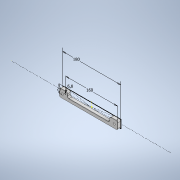
# Autodesk Inventor part: DisplayHolder
Saved by Autodesk Inventor 2022 (Build 260153000, 153)
## iProperties
Created: 2021-04-23
Part Number: DisplayHolder
Material: Generic
Document SubType Name: Modeling
Designer: Viktor
Density: 1 g/cm^3
Appearance: Default
Author: Viktor
## iProperties of the stored document DisplayHolder_3DPrint.ipt
Created: 2021-04-23
Part Number: DisplayHolder_3DPrint
Material: Generic
Document SubType Name: Modeling
Designer: Viktor
Density: 1 g/cm^3
Appearance: Default
Author: Viktor
Autodesk Inventor part; units mm, degrees
ref_plane "YZ Plane" through (0, 0, 0) normal (1, 0, 0) x (0, 1, 0)
ref_plane "XZ Plane" through (0, 0, 0) normal (0, 1, 0) x (-1, 0, 0)
ref_plane "XY Plane" through (0, 0, 0) normal (0, 0, 1) x (1, 0, 0)
sketch "Sketch1" plane through (0, 0, 0) normal (0, 0, 1) x (1, 0, 0)
  line L0 (-90, -12.5) -> (90, -12.5)
  line L1 (90, -12.5) -> (90, 12.5)
  line L2 (90, 12.5) -> (-90, 12.5)
  line L3 (-90, 12.5) -> (-90, -12.5)
  line L4 (-90, -12.5) -> (90, 12.5) construction
  line L5 (90, -12.5) -> (-90, 12.5) construction
  line L6 (-246.96, 0) -> (246.96, 0) construction
  circle A0 centre (-80, 0) radius 2.9
  line L7 (0, 17.5) -> (0, -17.5) construction
  line L8 (246.96, 0) -> (-246.96, 0) construction
  circle A1 centre (80, 0) radius 2.9
  point P0 (0, 0)
  dimension "d0" = 25
  dimension "d1" = 180
  dimension "d2" = 5.8
  dimension "d3" = 160
  constraints: 14 end point, 3 symmetric about line, 2 centre point, 2 midpoint, 2 parallel, 2 point on line, 1 horizontal, 1 perpendicular, 1 other
  measures "d0" distance between parallel lines of L0 L2
  measures "d1" distance of L1.end L2.end
  measures "d2" diameter of A0
  measures "d3" distance of A1.centre A0.centre
extrude "Extrusion1" add sketch "Sketch1" along normal blind 10
sketch "Sketch2" plane through (0, 0, 10) normal (0, 0, 1) x (1, 0, 0)
  line L0 (90, 12.5) -> (-90, 12.5) projected
  line L1 (-65, 12.5) -> (65, 12.5)
  line L2 (65, 12.5) -> (65, -2.5)
  line L3 (65, -2.5) -> (-65, -2.5)
  line L4 (-65, -2.5) -> (-65, 12.5)
  line L5 (-90, 12.5) -> (-90, -12.5) projected
  line L6 (90, -12.5) -> (90, 12.5) projected
  line L7 (-90, -12.5) -> (90, -12.5) projected
  point P0 (0, 0)
  dimension "d6" = 25
  dimension "d7" = 25
  dimension "d8" = 10
  constraints: 8 end point, 2 parallel, 1 horizontal, 1 perpendicular, 1 point on line
  measures "d6" distance between parallel lines of L5 L4
  measures "d7" distance between parallel lines of L6 L2
  measures "d8" distance between parallel lines of L7 L3
extrude "Extrusion2" cut sketch "Sketch2" against normal through all contours L2 L3 L4 L0
fillet "Fillet1" radius 5 8 edges at (-65, -2.5, 5) (-65, 12.5, 5) (-90, 12.5, 5) (-90, -12.5, 5) (90, -12.5, 5) (90, 12.5, 5) (65, 12.5, 5) (65, -2.5, 5)
chamfer "Chamfer1" distance 0.8 angle 45 32 edges at (0, -2.5, 0) (63.5355, -1.0355, 0) (65, 5, 0) (66.4645, 11.0355, 0) (77.5, 12.5, 0) (88.5355, 11.0355, 0) (90, 0, 0) (88.5355, -11.0355, 0) (0, -12.5, 0) (-88.5355, -11.0355, 0) (-90, 0, 0) (-88.5355, 11.0355, 0) (-77.5, 12.5, 0) (-66.4645, 11.0355, 0) (-65, 5, 0) (-63.5355, -1.0355, 0) (0, -2.5, 10) (-63.5355, -1.0355, 10) (-65, 5, 10) (-66.4645, 11.0355, 10) (-77.5, 12.5, 10) (-88.5355, 11.0355, 10) (-90, 0, 10) (-88.5355, -11.0355, 10) (0, -12.5, 10) (88.5355, -11.0355, 10) (90, 0, 10) (88.5355, 11.0355, 10) (77.5, 12.5, 10) (66.4645, 11.0355, 10) (65, 5, 10) (63.5355, -1.0355, 10)
body "Solid1"
